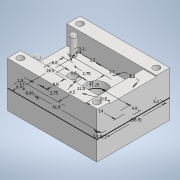
# Autodesk Inventor part: motor holder under
Saved by Autodesk Inventor 2022 (Build 260153000, 153)
## iProperties
Created: 2021-11-29
Part Number: motor holder under
Material: Generic
Document SubType Name: Modeling
Designer: Alec Warren
Density: 1 g/cm^3
Appearance: Default
Author: Alec Warren
Autodesk Inventor part; units mm, degrees
ref_plane "YZ Plane" through (0, 0, 0) normal (1, 0, 0) x (0, 1, 0)
ref_plane "XZ Plane" through (0, 0, 0) normal (0, 1, 0) x (-1, 0, 0)
ref_plane "XY Plane" through (0, 0, 0) normal (0, 0, 1) x (1, 0, 0)
sketch "Sketch1" plane through (0, 0, 0) normal (0, 1, 0) x (-1, 0, 0)
  line L0 (0, 0) -> (0, 22.5)
  line L1 (0, 22.5) -> (-41.8, 22.5)
  line L2 (-41.8, 22.5) -> (-41.8, 0)
  line L3 (-41.8, 0) -> (0, 0)
  line L4 (0, 11.25) -> (-37, 11.25)
  line L5 (-37, 11.25) -> (-41.8, 11.25)
  line L6 (-39.4, 11.25) -> (-25.4, 11.25)
  line L7 (-25.4, 11.25) -> (-14.15, 11.25)
  line L8 (-14.15, 11.25) -> (-5.55, 11.25)
  line L9 (-5.55, 11.25) -> (-5.55, 2.45)
  line L10 (-5.55, 11.25) -> (-5.55, 20.05)
  circle A0 centre (-5.55, 2.45) radius 1.375
  circle A1 centre (-5.55, 20.05) radius 1.375
  line L11 (-37, 0) -> (-37, 22.5)
  line L12 (0, 22.5) -> (0, 28.9)
  line L13 (0, 0) -> (0, -6.4)
  line L14 (0, -6.4) -> (-41.8, -6.4)
  line L15 (-41.8, -6.4) -> (-41.8, 0)
  line L16 (-41.8, 22.5) -> (-41.8, 28.9)
  line L17 (-41.8, 28.9) -> (0, 28.9)
  line L18 (0, -3.2) -> (-3.2, -3.2)
  line L19 (0, 25.7) -> (-3.2, 25.7)
  circle A2 centre (-3.2, -3.2) radius 1.6
  circle A3 centre (-25.4, 11.25) radius 5.25
  line L20 (-38.6, -3.2) -> (-3.2, -3.2)
  line L21 (-3.2, -3.2) -> (-20.9, -3.2)
  circle A4 centre (-12.05, -3.2) radius 1.6
  line L22 (-38.6, -3.2) -> (-20.9, -3.2)
  circle A5 centre (-20.9, -3.2) radius 1.6
  circle A6 centre (-29.75, -3.2) radius 1.6
  circle A7 centre (-3.2, 25.7) radius 1.6
  circle A8 centre (-14.15, 11.25) radius 2.25
  circle A9 centre (-3.2, 25.7) radius 1.45
  line L23 (-41.8, 25.7) -> (-41.8, -3.2)
  circle A10 centre (-12.05, 25.7) radius 1.45
  circle A11 centre (-20.9, 25.7) radius 1.45
  circle A12 centre (-29.75, 25.7) radius 1.45
  circle A13 centre (-38.6, 25.7) radius 1.45
  circle A14 centre (-3.2, -3.2) radius 1.45
  circle A15 centre (-12.05, -3.2) radius 1.45
  circle A16 centre (-20.9, -3.2) radius 1.45
  circle A17 centre (-29.75, -3.2) radius 1.45
  circle A18 centre (-38.6, -3.2) radius 1.45
  line L24 (-41.8, 28.9) -> (-43.4, 28.9)
  line L25 (-43.4, 28.9) -> (-43.4, -6.4)
  line L26 (-43.4, -6.4) -> (-41.8, -6.4)
  line L27 (-41.8, 22.5) -> (-43.4, 22.5)
  line L28 (-41.8, 0) -> (-43.4, 0)
  line L29 (-43.4, -3.2) -> (-40.2, -3.2)
  circle A19 centre (-40.2, -3.2) radius 1.6
  line L30 (-43.4, 25.7) -> (-40.2, 25.7)
  circle A20 centre (-40.2, 25.7) radius 1.6
  dimension "d0" = 22.5
  dimension "d1" = 41.8
  dimension "d2" = 37
  dimension "d3" = 4.8
  dimension "d4" = 14
  dimension "d5" = 11.25
  dimension "d6" = 8.6
  dimension "d7" = 8.8
  dimension "d8" = 8.8
  dimension "d9" = 2.75
  dimension "d10" = 2.75
  dimension "d12" = 6.4
  dimension "d13" = 6.4
  dimension "d15" = 3.2
  dimension "d18" = 3.2
  dimension "d19" = 3.2
  dimension "d23" = 10.5
  dimension "d24" = 3.2
  dimension "d25" = 3.2
  dimension "d26" = 3.2
  dimension "d35" = 4.5
  dimension "d36" = 2.9
  dimension "d37" = 28.9
  dimension "d40" = 8.85
  dimension "d43" = 28.9
  dimension "d53" = 1.6
  dimension "d58" = 3.2
  dimension "d59" = 3.2
  dimension "d60" = 3.2
  constraints: 62 end point, 21 centre point, 11 perpendicular, 10 midpoint, 10 point on line, 9 coincident, 7 horizontal, 6 vertical, 1 collinear, 1 symmetric about line, 18 other
  measures "d0" distance of L0.start L0.end
  measures "d1" distance of L0.end L1.end
  measures "d2" distance of L4.start L4.end
  measures "d3" distance of L4.end L5.end
  measures "d4" distance of L6.start L6.end
  measures "d5" distance of L6.end L7.end
  measures "d6" distance of L7.end L8.end
  measures "d7" distance of L8.end L9.end
  measures "d8" distance of L8.end L10.end
  measures "d9" diameter of A0
  measures "d10" diameter of A1
  measures "d12" distance of L0.end L12.end
  measures "d13" distance of L0.start L13.end
  measures "d15" distance of L18.start L18.end
  measures "d18" distance of L19.start L19.end
  measures "d19" diameter of A2
  measures "d23" diameter of A3
  measures "d24" diameter of A4
  measures "d25" diameter of A5
  measures "d26" diameter of A6
  measures "d35" diameter of A8
  measures "d36" diameter of A9
  measures "d37" distance of L23.start L23.end
  measures "d40" distance of A9.centre A10.centre
  measures "d43" distance of A9.centre A14.centre
  measures "d53" distance of L16.end L24.end
  measures "d58" distance of L29.start L29.end
  measures "d59" distance of L30.start L30.end
  measures "d60" diameter of A20
extrude "Extrusion1" add sketch "Sketch1" along normal blind 3.2 contours L3 L11 L4 A3 A8 L0 | L13 L18 A2 L20 A4 A5 A6 A18 A19 L15 L3 | L4 A8 A3 L11 L1 L0 | L3 L2 L5 L11 | L13 L14 L15 A19 A18 L20 A6 A5 A4 A2 L18 | A20 A13 | L1 L16 L17 L12 | L28 L25 L27 L2 | L15 L29 L25 L28 | L5 L2 L1 L11 | A2 L20 A14 L18 | L18 A14 L20 A2 | L15 L26 L25 L29 | A19 A18 | A14 L20 L18 | L18 L20 A14 | L27 L25 L30 L16 | A19 A18 | A18 L20 A19 | A19 L20 A18 | A4 L20 A15 | L20 A15 A4 | L30 L25 L24 L16 | A15 L20 | L20 A15 | A20 A13 | A13 A20 | A6 L20 A17 | L20 A17 A6 | A5 L20 A16 | L20 A16 A5 | A17 L20 | L20 A17 | A16 L20 | L20 A16 | A0 | A1 | A7 | A9 | A10 | A11 | A12
extrude "Extrusion2" add sketch "Sketch1" along normal blind 9.3 from surface at 3.2 contours L13 L18 A2 L20 A4 A5 A6 A18 A19 L15 L3 | L13 L14 L15 A19 A18 L20 A6 A5 A4 A2 L18 | A20 A13 | L1 L16 L17 L12 | A2 L20 A14 L18 | L18 A14 L20 A2 | A19 A18 | A14 L20 L18 | L18 L20 A14 | A19 A18 | A18 L20 A19 | A19 L20 A18 | A4 L20 A15 | L20 A15 A4 | A15 L20 | L20 A15 | A20 A13 | A13 A20 | A6 L20 A17 | L20 A17 A6 | A5 L20 A16 | L20 A16 A5 | A17 L20 | L20 A17 | A16 L20 | L20 A16 | A0 | A1 | A7 | A9 | A10 | A11 | A12
extrude "Extrusion4" add sketch "Sketch1" along normal blind 8.7 from surface at 3.2 contours L3 L2 L5 L11 | L5 L2 L1 L11
fillet "Fillet2" radius 1.35 2 edges at (6.925, 12.5, 2.45) (6.925, 12.5, 20.05)
extrude "Extrusion6" add sketch "Sketch1" against normal blind 9.5 contours L3 L11 L4 A3 A8 L0 | L13 L18 A2 L20 A4 A5 A6 A18 A19 L15 L3 | L4 A8 A3 L11 L1 L0 | L3 L2 L5 L11 | L13 L14 L15 A19 A18 L20 A6 A5 A4 A2 L18 | A20 A13 | L1 L16 L17 L12 | L28 L25 L27 L2 | L15 L29 L25 L28 | L5 L2 L1 L11 | A2 L20 A14 L18 | L18 A14 L20 A2 | A8 L4 | L4 A8 | L15 L26 L25 L29 | A19 A18 | A14 L20 L18 | L18 L20 A14 | L27 L25 L30 L16 | A19 A18 | A18 L20 A19 | A19 L20 A18 | A4 L20 A15 | L20 A15 A4 | L30 L25 L24 L16 | A15 L20 | L20 A15 | A20 A13 | A13 A20 | A6 L20 A17 | L20 A17 A6 | A5 L20 A16 | L20 A16 A5 | A17 L20 | L20 A17 | A16 L20 | L20 A16 | A0 | A1 | A7 | A9 | A10 | A11 | A12
extrude "Extrusion7" add sketch "Sketch1" along normal up to surface (12.5 mm away) contours L15 L29 L25 L28 | L15 L26 L25 L29 | L27 L25 L30 L16 | L30 L25 L24 L16
extrude "Extrusion8" add sketch "Sketch1" along normal up to surface (11.9 mm away) contours L28 L25 L27 L2
extrude "Extrusion9" cut sketch "Sketch1" against normal blind 10 from surface at 12.5 contours A20 A13 | A2 L20 A14 L18 | L18 A14 L20 A2 | A19 A18 | A14 L20 L18 | L18 L20 A14 | A19 A18 | A20 A13 | A7 | A9 picked at (-41.1972, 25.8881) picked at (-39.0944, 25.8832)
body "Solid1"
